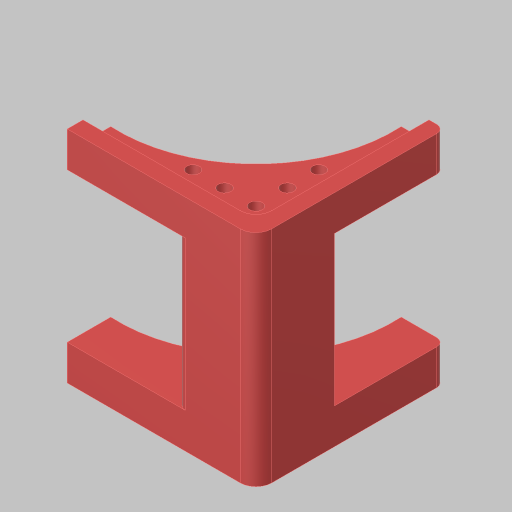
# Autodesk Inventor part: DB1-016
Saved by Autodesk Inventor 2023.5 (Build 275446000, 446)
## iProperties
Created: 2025-03-03
Part Number: DB1-016
Material: ABS Plastic
Document SubType Name: Modeling
Designer: AIM
Density: 1.06 g/cm^3
Appearance: Smooth - Red
Author: AIM
Autodesk Inventor part; units mm, degrees
ref_plane "YZ Plane" through (0, 0, 0) normal (1, 0, 0) x (0, 1, 0)
ref_plane "XZ Plane" through (0, 0, 0) normal (0, 1, 0) x (-1, 0, 0)
ref_plane "XY Plane" through (0, 0, 0) normal (0, 0, 1) x (1, 0, 0)
sketch "Sketch2" plane through (0, 0, 0) normal (0, 1, 0) x (-1, 0, 0)
  line L0 (15.875, -15.875) -> (-15.875, -15.875)
  line L1 (-15.875, -15.875) -> (-15.875, 15.875)
  line L2 (-15.875, 15.875) -> (15.875, 15.875)
  line L3 (15.875, 15.875) -> (15.875, -15.875)
  line L4 (15.875, -15.875) -> (-15.875, 15.875) construction
  line L5 (-15.875, -15.875) -> (15.875, 15.875) construction
  point P0 (0, 0)
  dimension "d0" = 31.75
  dimension "d1" = 31.75
  constraints: 12 end point, 2 midpoint, 2 parallel, 1 horizontal, 1 perpendicular
  measures "d0" distance of L1.end L2.end
  measures "d1" distance of L0.end L1.end
extrude "Extrusion1" add sketch "Sketch2" along normal blind 76.1492
sketch "Sketch3" plane through (0, 0, 0) normal (0, -1, 0) x (1, 0, 0)
  circle A0 centre (-3.175, -3.175) radius 3.9688
  line L0 (15.875, -15.875) -> (-15.875, -15.875) projected
  line L1 (-15.875, -15.875) -> (-15.875, 15.875) projected
  line L2 (-15.875, 9.1217) -> (3.175, 9.1217)
  line L3 (9.525, 2.7717) -> (9.525, -15.875)
  arc A1 (9.525, 2.7717) -> (3.175, 9.1217) centre (3.175, 2.7717) ccw
  line L4 (-15.875, -15.875) -> (-15.875, 15.875) projected
  line L5 (-15.875, 15.875) -> (15.875, 15.875) projected
  line L6 (15.875, 15.875) -> (15.875, -15.875) projected
  line L7 (15.875, -15.875) -> (-15.875, -15.875) projected
  point P0 (-6.35, 9.1217)
  dimension "d4" = 7.9375
  dimension "d6" = 12.7
  dimension "d7" = 12.7
  dimension "d8" = 12.7
  dimension "d9" = 12.7
  dimension "d10" = 6.35
  constraints: 4 end point, 2 centre point, 2 point on circle, 2 point on line, 2 tangent, 1 coincident, 1 horizontal, 1 midpoint, 1 perpendicular
  measures "d4" diameter of A0
  measures "d6" distance from line of L1 point (-3.175, -3.175)
  measures "d7" distance from line of L0 point (-3.175, -3.175)
  measures "d8" distance from line of L3 point (-3.175, -3.175)
  measures "d9" distance of point (-6.35, 9.122) point (-3.175, -3.175)
  measures "d10" radius of A1
extrude "Extrusion2" add sketch "Sketch3" along normal blind 7.9375 contours L0 L3 A1 L2 L1 L5 L6
sketch "Sketch4" plane through (0, 76.1492, 0) normal (0, 1, 0) x (1, 0, 0)
  line L0 (15.875, 15.875) -> (-15.875, 15.875) projected
  line L1 (-15.875, -15.875) -> (-15.875, 15.875) projected
  line L2 (-15.875, 15.875) -> (15.875, 15.875) projected
  line L3 (15.875, 15.875) -> (15.875, -15.875) projected
  line L4 (15.875, -15.875) -> (-15.875, -15.875) projected
  line L5 (9.525, 15.875) -> (-15.875, 15.875) projected
  line L6 (9.525, 15.875) -> (9.525, -3.175)
  line L7 (3.175, -9.525) -> (-15.875, -9.525)
  line L8 (-15.875, 15.875) -> (-15.875, -9.1217) projected
  arc A0 (3.175, -9.525) -> (9.525, -3.175) centre (3.175, -3.175) ccw
  line L9 (6.35, 15.875) -> (6.35, -3.175)
  arc A1 (3.175, -6.35) -> (6.35, -3.175) centre (3.175, -3.175) ccw
  line L10 (3.175, -6.35) -> (-15.875, -6.35)
  point P0 (0, 0)
  point P1 (-3.175, 3.175)
  dimension "d13" = 12.7
  dimension "d14" = 12.7
  dimension "d15" = 12.7
  dimension "d16" = 12.7
  dimension "d17" = 6.35
  dimension "d20" = 3.175
  constraints: 8 end point, 4 point on circle, 2 centre point, 2 point on line, 2 tangent, 1 perpendicular, 1 vertical, 2 other
  measures "d13" distance from line of L0 point (-3.175, 3.175)
  measures "d14" distance from line of L1 point (-3.175, 3.175)
  measures "d15" distance from line of point (-3.175, 3.175) L7
  measures "d16" distance from line of L6 point (-3.175, 3.175)
  measures "d17" radius of A0
  measures "d20" radial gap between concentric circles of A0 A1
extrude "Extrusion3" add sketch "Sketch4" along normal blind 4.7625 contours L3 L4 L1 L7 A0 L6 L0
extrude "Extrusion4" cut sketch "Sketch4" against normal blind 3.175 contours L9 A1 L10 L1 L0
sketch "Sketch5" plane through (9.525, 0, -15.875) normal (0, 0, -1) x (-1, 0, 0)
  line L0 (0, 0) -> (0, -7.9375) projected
  line L1 (0, -7.9375) -> (-6.35, -7.9375) projected
  line L2 (-6.35, -7.9375) -> (-6.35, 80.9117) projected
  line L3 (-6.35, 80.9117) -> (0, 80.9117) projected
  line L4 (0, 80.9117) -> (0, 76.1492) projected
  line L5 (0, 76.1492) -> (3.175, 76.1492) projected
  line L6 (3.175, 76.1492) -> (3.175, 72.9742) projected
  line L7 (3.175, 72.9742) -> (25.4, 72.9742) projected
  line L8 (25.4, 72.9742) -> (25.4, 0) projected
  line L9 (25.4, 0) -> (0, 0) projected
  line L10 (-6.35, 66.6242) -> (25.4, 66.6242)
  line L11 (16.9333, 66.6242) -> (16.9333, 72.9742)
  line L12 (25.4, 0) -> (25.4, 72.9742) projected
  line L13 (25.4, 6.35) -> (-6.35, 6.35)
  point P0 (9.525, 0)
  dimension "d23" = 6.35
  dimension "d53" = 8.4667
  dimension "d60" = 6.35
  constraints: 6 end point, 6 point on line, 2 perpendicular, 1 vertical
  measures "d23" distance between parallel lines of L7 L10
  measures "d53" distance between parallel lines of L8 L11
  measures "d60" distance between parallel lines of L9 L13
extrude "Extrusion6" add sketch "Sketch5" along normal blind 44.45 contours L0 L1 L2 L13 L8 L9 | L10 L11 L7 L8 | L2 L3 L4 L5 L6 L7 L11 L10
sketch "Sketch6" plane through (-15.875, 0, -15.875) normal (-1, 0, 0) x (0, 0, 1)
  line L0 (24.9967, -7.9375) -> (24.9967, 0) projected
  line L1 (-44.45, 72.9742) -> (22.225, 72.9742) projected
  line L2 (22.225, 72.9742) -> (22.225, 76.1492) projected
  line L3 (22.225, 76.1492) -> (25.4, 76.1492) projected
  line L4 (25.4, 76.1492) -> (25.4, 80.9117) projected
  line L5 (25.4, 80.9117) -> (31.75, 80.9117) projected
  line L6 (31.75, 80.9117) -> (31.75, -7.9375) projected
  line L7 (31.75, -7.9375) -> (24.9967, -7.9375) projected
  line L8 (0, -7.9375) -> (0, 80.9117) projected
  line L9 (0, 66.6242) -> (31.75, 66.6242)
  line L10 (31.75, -7.9375) -> (31.75, 80.9117) projected
  line L11 (8.4667, 66.6242) -> (8.4667, 72.9742)
  line L12 (0, 6.35) -> (31.75, 6.35)
  line L13 (24.9967, 0) -> (-44.45, 0) projected
  line L14 (-44.45, 0) -> (-44.45, 6.35) projected
  line L15 (-44.45, 6.35) -> (0, 6.35) projected
  line L16 (0, 6.35) -> (0, 66.6242) projected
  line L17 (0, 66.6242) -> (-44.45, 66.6242) projected
  line L18 (-44.45, 66.6242) -> (-44.45, 72.9742) projected
  point P0 (15.875, 0)
  point P1 (0, 0)
  point P2 (0, 72.9742)
  point P3 (31.75, 66.6242)
  dimension "d24" = 6.35
  constraints: 6 end point, 6 point on line, 3 perpendicular
  measures "d24" distance between parallel lines of L1 L9
extrude "Extrusion5" add sketch "Sketch6" along normal blind 44.45 contours L0 L13 L8 L12 L6 L7 | L13 L14 L15 L8 | L9 L11 L1 L2 L3 L4 L5 L6 | L17 L18 L1 L8 | L8 L1 L11 L9
sketch "Sketch9" plane through (0, 72.9742, 0) normal (0, 1, 0) x (1, 0, 0)
  line L0 (3.175, -6.35) -> (-60.325, -6.35) projected
  line L1 (6.35, 60.325) -> (6.35, -3.175) projected
  line L2 (3.175, -9.525) -> (-60.325, -9.525) projected
  line L3 (9.525, -3.175) -> (9.525, 60.325) projected
  point P0 (0, 0)
  point P1 (-3.175, 3.175)
  point P2 (-15.875, 3.175)
  point P3 (-28.575, 3.175)
  point P4 (-3.175, 15.875)
  point P5 (-3.175, 28.575)
  dimension "d35" = 12.7
  dimension "d36" = 12.7
  dimension "d37" = 12.7
  dimension "d38" = 12.7
  dimension "d39" = 12.7
  dimension "d40" = 12.7
  constraints: 2 horizontal alignment, 2 vertical alignment
  measures "d35" distance of point (-3.175, 3.175) point (-3.175, 15.875)
  measures "d36" distance of point (-3.175, 28.575) point (-3.175, 15.875)
  measures "d37" distance of point (-15.875, 3.175) point (-3.175, 3.175)
  measures "d38" distance of point (-28.575, 3.175) point (-15.875, 3.175)
  measures "d39" distance from line of point (-3.175, 3.175) L2
  measures "d40" distance from line of L3 point (-3.175, 3.175)
fillet "Fillet2" radius 6.35 2 edges at (15.875, 36.4871, 15.875) (-15.875, 36.4871, -15.875)
hole "Hole1" at (-3.175, 72.9742, -3.175) at (-15.875, 72.9742, -3.175) at (-28.575, 72.9742, -3.175) at (-3.175, 72.9742, -15.875) at (-3.175, 72.9742, -28.575) direction (0, -1, 0) diameter 5.1054 end through all clearance for "Flat Head Machine Screw (82)" size "#10" standard "Ansi Unified Screw Threads"
sketch "Sketch11" plane through (0, 72.9742, 0) normal (0, 1, 0) x (1, 0, 0)
  line L0 (-11.6417, 60.325) -> (-11.6417, 11.6417)
  line L1 (-11.6417, 11.6417) -> (-60.325, 11.6417)
  line L2 (-60.325, 60.325) -> (-60.325, -15.875) projected
  circle A0 centre (-28.575, 3.175) radius 2.5527 projected
  circle A1 centre (-3.175, 28.575) radius 2.5527 projected
  circle A2 centre (-3.175, 15.875) radius 2.5527 projected
  circle A3 centre (-15.875, 3.175) radius 2.5527 projected
  circle A4 centre (-3.175, 3.175) radius 2.5527 projected
  circle A5 centre (-28.575, 3.175) radius 2.5527 projected
  circle A6 centre (-3.175, 28.575) radius 2.5527 projected
  line L3 (-60.325, -15.875) -> (-60.325, -6.35) projected
  line L4 (-60.325, -6.35) -> (-60.325, 60.325) projected
  line L5 (6.35, -3.175) -> (6.35, 60.325) projected
  arc A7 (3.175, -6.35) -> (6.35, -3.175) centre (3.175, -3.175) ccw projected
  line L6 (-60.325, -6.35) -> (3.175, -6.35) projected
  line L7 (9.525, -15.875) -> (-60.325, -15.875) projected
  arc A8 (9.525, -15.875) -> (15.875, -9.525) centre (9.525, -9.525) ccw projected
  line L8 (15.875, 60.325) -> (15.875, -9.525) projected
  line L9 (6.35, 60.325) -> (15.875, 60.325) projected
  line L10 (-60.325, 60.325) -> (6.35, 60.325) projected
  point P0 (0, 0)
  point P1 (-60.325, 15.875)
  point P2 (-15.875, 60.325)
  dimension "d54" = 8.4667
  dimension "d55" = 8.4667
  constraints: 4 end point, 1 perpendicular, 1 point on line, 1 vertical
  measures "d54" distance from line of A0.centre L1
  measures "d55" distance from line of A1.centre L0
extrude "Extrusion9" [suppressed]
sketch "Sketch12" plane through (0, 0, 0) normal (0, 1, 0) x (-1, 0, 0)
  circle A0 centre (57.15, -57.15) radius 55.5625
  circle A1 centre (3.175, -3.175) radius 2.5527 projected
  point P0 (0, 0)
  dimension "d62" = 53.975
  dimension "d63" = 53.975
  dimension "d64" = 111.125
  constraints: 1 centre point
  measures "d62" horizontal distance of A1.centre A0.centre
  measures "d63" horizontal distance of A1.centre A0.centre
  measures "d64" diameter of A0
loft "Loft1" [suppressed]
loft "Loft2" [suppressed]
extrude "Extrusion11" cut sketch "Sketch12" along normal through all both and the other way through all contours A0
fillet "Fillet7" radius 3.175 3 edges at (-15.875, 36.4871, 15.875) (15.875, 73.7679, -60.325) (15.875, -0.7938, -60.325)
body "Solid1"
